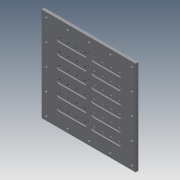
# Autodesk Inventor part: plate
Saved by Autodesk Inventor 2016 (Build 200138000, 138)
## iProperties
Created: 2013-02-21
Part Number: plate
Material: Generic
Document SubType Name: Modeling
Designer: Dave
Density: 1 g/cm^3
Appearance: Default
Author: Dave
Autodesk Inventor part; units mm, degrees
ref_plane "YZ Plane" through (0, 0, 0) normal (1, 0, 0) x (0, 1, 0)
ref_plane "XZ Plane" through (0, 0, 0) normal (0, 1, 0) x (-1, 0, 0)
ref_plane "XY Plane" through (0, 0, 0) normal (0, 0, 1) x (1, 0, 0)
sketch "Sketch1" plane through (0, 0, 0) normal (0, 0, 1) x (1, 0, 0)
  line L0 (0, 0) -> (219.964, 0)
  line L1 (219.964, 0) -> (219.964, 219.964)
  line L2 (219.964, 219.964) -> (0, 219.964)
  line L3 (0, 219.964) -> (0, 0)
  dimension "d0" = 219.964
  dimension "d1" = 219.964
  constraints: 8 end point, 2 parallel, 1 horizontal, 1 perpendicular
  measures "d0" distance of L0.start L0.end
  measures "d1" distance of L2.end L0.start
extrude "Plate" add sketch "Sketch1" along normal blind 6.5532
sketch "Sketch6" plane through (0, 0, 6.5532) normal (0, 0, 1) x (1, 0, 0)
  line L0 (0, 0) -> (0, 219.964) projected
  line L1 (219.964, 0) -> (0, 0) projected
  line L2 (219.964, 219.964) -> (219.964, 0) projected
  line L3 (0, 219.964) -> (219.964, 219.964) projected
  circle A0 centre (10.16, 209.804) radius 4.421
  circle A1 centre (60.071, 209.804) radius 4.421
  circle A2 centre (109.982, 209.804) radius 4.421
  circle A3 centre (159.893, 209.804) radius 4.421
  circle A4 centre (209.804, 209.804) radius 4.421
  circle A5 centre (10.16, 159.893) radius 4.421
  circle A6 centre (10.16, 109.982) radius 4.421
  circle A7 centre (10.16, 60.071) radius 4.421
  circle A8 centre (10.16, 10.16) radius 4.421
  circle A9 centre (60.071, 10.16) radius 4.421
  circle A10 centre (109.982, 10.16) radius 4.421
  circle A11 centre (159.893, 10.16) radius 4.421
  circle A12 centre (209.804, 10.16) radius 4.421
  circle A13 centre (209.804, 159.893) radius 4.421
  circle A14 centre (209.804, 109.982) radius 4.421
  circle A15 centre (209.804, 60.071) radius 4.421
  circle A16 centre (209.804, 10.16) radius 4.421
  dimension "d56" = 10.16
  dimension "d58" = 10.16
  dimension "d61" = 49.911
  dimension "d68" = 49.911
  dimension "d75" = 49.911
  dimension "d82" = 49.911
  constraints: 17 centre point, 2 horizontal, 2 vertical, 32 other
  measures "d56" distance from line of A0.centre L3
  measures "d58" distance from line of A0.centre L0
  measures "d61" distance of A0.centre A1.centre
  measures "d68" distance of A0.centre A5.centre
  measures "d75" distance of A8.centre A9.centre
  measures "d82" distance of A4.centre A13.centre
hole "Boundary" at (10.16, 209.804, 6.5532) at (60.071, 209.804, 6.5532) at (10.16, 159.893, 6.5532) at (109.982, 209.804, 6.5532) at (10.16, 109.982, 6.5532) at (159.893, 209.804, 6.5532) at (10.16, 60.071, 6.5532) at (209.804, 209.804, 6.5532) at (10.16, 10.16, 6.5532) at (209.804, 159.893, 6.5532) at (60.071, 10.16, 6.5532) at (209.804, 109.982, 6.5532) at (109.982, 10.16, 6.5532) at (209.804, 60.071, 6.5532) at (159.893, 10.16, 6.5532) at (209.804, 10.16, 6.5532) direction (0, 0, -1) diameter 6.35 end through all
sketch "Sketch10" plane through (0, 0, 6.5532) normal (0, 0, 1) x (1, 0, 0)
  circle A0 centre (10.16, 209.804) radius 3.175 projected
  line L0 (0, 0) -> (0, 219.964) projected
  line L1 (0, 219.964) -> (219.964, 219.964) projected
  circle A1 centre (40.4114, 179.5526) radius 3.175
  circle A2 centre (60.4012, 179.5526) radius 3.175
  circle A3 centre (80.391, 179.5526) radius 3.175
  circle A4 centre (100.3808, 179.5526) radius 3.175
  circle A5 centre (120.3706, 179.5526) radius 3.175
  circle A6 centre (140.3604, 179.5526) radius 3.175
  circle A7 centre (160.3502, 179.5526) radius 3.175
  circle A8 centre (180.34, 179.5526) radius 3.175
  circle A9 centre (40.4114, 151.5618) radius 3.175
  circle A10 centre (60.4012, 151.5618) radius 3.175
  circle A11 centre (80.391, 151.5618) radius 3.175
  circle A12 centre (100.3808, 151.5618) radius 3.175
  circle A13 centre (120.3706, 151.5618) radius 3.175
  circle A14 centre (140.3604, 151.5618) radius 3.175
  circle A15 centre (160.3502, 151.5618) radius 3.175
  circle A16 centre (180.34, 151.5618) radius 3.175
  circle A17 centre (40.4114, 123.571) radius 3.175
  circle A18 centre (60.4012, 123.571) radius 3.175
  circle A19 centre (80.391, 123.571) radius 3.175
  circle A20 centre (100.3808, 123.571) radius 3.175
  circle A21 centre (120.3706, 123.571) radius 3.175
  circle A22 centre (140.3604, 123.571) radius 3.175
  circle A23 centre (160.3502, 123.571) radius 3.175
  circle A24 centre (180.34, 123.571) radius 3.175
  circle A25 centre (40.4114, 95.5802) radius 3.175
  circle A26 centre (60.4012, 95.5802) radius 3.175
  circle A27 centre (80.391, 95.5802) radius 3.175
  circle A28 centre (100.3808, 95.5802) radius 3.175
  circle A29 centre (120.3706, 95.5802) radius 3.175
  circle A30 centre (140.3604, 95.5802) radius 3.175
  circle A31 centre (160.3502, 95.5802) radius 3.175
  circle A32 centre (180.34, 95.5802) radius 3.175
  circle A33 centre (40.4114, 67.5894) radius 3.175
  circle A34 centre (60.4012, 67.5894) radius 3.175
  circle A35 centre (80.391, 67.5894) radius 3.175
  circle A36 centre (100.3808, 67.5894) radius 3.175
  circle A37 centre (120.3706, 67.5894) radius 3.175
  circle A38 centre (140.3604, 67.5894) radius 3.175
  circle A39 centre (160.3502, 67.5894) radius 3.175
  circle A40 centre (180.34, 67.5894) radius 3.175
  circle A41 centre (40.4114, 39.5986) radius 3.175
  circle A42 centre (60.4012, 39.5986) radius 3.175
  circle A43 centre (80.391, 39.5986) radius 3.175
  circle A44 centre (100.3808, 39.5986) radius 3.175
  circle A45 centre (120.3706, 39.5986) radius 3.175
  circle A46 centre (140.3604, 39.5986) radius 3.175
  circle A47 centre (160.3502, 39.5986) radius 3.175
  circle A48 centre (180.34, 39.5986) radius 3.175
  dimension "d175" = 6.35
  dimension "d177" = 30.2514
  dimension "d178" = 30.2514
  dimension "d181" = 19.9898
  dimension "d184" = 27.9908
  constraints: 48 centre point, 1 horizontal, 1 vertical, 94 other
  measures "d175" diameter of A1
  measures "d177" horizontal distance of A0.centre A1.centre
  measures "d178" horizontal distance of A1.centre A0.centre
  measures "d181" distance of A1.centre A2.centre
  measures "d184" distance of A1.centre A9.centre
hole "SMA" at (80.391, 123.571, 6.5532) at (100.3808, 123.571, 6.5532) at (80.391, 151.5618, 6.5532) at (100.3808, 151.5618, 6.5532) at (80.391, 179.5526, 6.5532) at (100.3808, 179.5526, 6.5532) at (60.4012, 151.5618, 6.5532) at (40.4114, 151.5618, 6.5532) at (40.4114, 179.5526, 6.5532) at (60.4012, 179.5526, 6.5532) at (40.4114, 123.571, 6.5532) at (60.4012, 123.571, 6.5532) at (40.4114, 95.5802, 6.5532) at (60.4012, 95.5802, 6.5532) at (80.391, 95.5802, 6.5532) at (100.3808, 67.5894, 6.5532) at (80.391, 67.5894, 6.5532) at (80.391, 39.5986, 6.5532) at (60.4012, 67.5894, 6.5532) at (60.4012, 39.5986, 6.5532) at (40.4114, 39.5986, 6.5532) at (40.4114, 67.5894, 6.5532) at (100.3808, 95.5802, 6.5532) at (120.3706, 179.5526, 6.5532) at (140.3604, 179.5526, 6.5532) at (160.3502, 179.5526, 6.5532) at (180.34, 179.5526, 6.5532) at (120.3706, 151.5618, 6.5532) at (140.3604, 151.5618, 6.5532) at (120.3706, 95.5802, 6.5532) at (140.3604, 123.571, 6.5532) at (140.3604, 95.5802, 6.5532) at (160.3502, 151.5618, 6.5532) at (160.3502, 123.571, 6.5532) at (180.34, 151.5618, 6.5532) at (160.3502, 95.5802, 6.5532) at (180.34, 123.571, 6.5532) at (180.34, 95.5802, 6.5532) at (120.3706, 123.571, 6.5532) at (100.3808, 39.5986, 6.5532) at (120.3706, 67.5894, 6.5532) at (120.3706, 39.5986, 6.5532) at (140.3604, 67.5894, 6.5532) at (140.3604, 39.5986, 6.5532) at (160.3502, 67.5894, 6.5532) at (160.3502, 39.5986, 6.5532) at (180.34, 67.5894, 6.5532) at (180.34, 39.5986, 6.5532) direction (0, 0, -1) diameter 5.588 end through all thread size "1/4-36 UNS" class "2B" standard "ANSI Unified Screw Threads"
sketch "Sketch12" plane through (0, 0, 6.5532) normal (0, 0, 1) x (1, 0, 0)
  circle A0 centre (40.4114, 179.5526) radius 2.794 projected
  circle A1 centre (80.391, 179.5526) radius 2.794 projected
  circle A2 centre (100.3808, 179.5526) radius 2.794 projected
  circle A3 centre (60.4012, 179.5526) radius 2.794 projected
  arc A4 (40.4114, 185.9026) -> (40.4114, 173.2026) centre (40.4114, 179.5526) ccw
  arc A5 (100.3808, 173.2026) -> (100.3808, 185.9026) centre (100.3808, 179.5526) ccw
  line L0 (40.4114, 185.9026) -> (100.3808, 185.9026)
  line L1 (40.4114, 173.2026) -> (100.3808, 173.2026)
  dimension "d211" = 12.7
  dimension "d213" = 12.7
  constraints: 4 end point, 4 point on circle, 2 centre point, 2 coincident, 2 tangent, 1 parallel
  measures "d211" diameter of A4
  measures "d213" diameter of A5
extrude "Extrusion3" cut sketch "Sketch12" against normal blind 2.667
pattern_linear "Rectangular Pattern1" count 2 spacing 80.01 along (1, 0, 0) count 6 spacing 27.9908 along (0, -1, 0) of "Extrusion3"
sketch "Sketch11" plane through (0, 0, 6.5532) normal (0, 0, 1) x (1, 0, 0)
  circle A0 centre (40.4114, 179.5526) radius 2.794 projected
  line L0 (0, 0) -> (0, 219.964) projected
  line L1 (0, 219.964) -> (219.964, 219.964) projected
  circle A1 centre (31.5214, 188.4426) radius 2.4311
  circle A2 centre (110.2614, 188.4426) radius 2.4311
  circle A3 centre (189.0014, 188.4426) radius 2.4311
  circle A4 centre (31.5214, 160.4518) radius 2.4311
  circle A5 centre (110.2614, 160.4518) radius 2.4311
  circle A6 centre (189.0014, 160.4518) radius 2.4311
  circle A7 centre (31.5214, 132.461) radius 2.4311
  circle A8 centre (110.2614, 132.461) radius 2.4311
  circle A9 centre (189.0014, 132.461) radius 2.4311
  circle A10 centre (31.5214, 104.4702) radius 2.4311
  circle A11 centre (110.2614, 104.4702) radius 2.4311
  circle A12 centre (189.0014, 104.4702) radius 2.4311
  circle A13 centre (31.5214, 76.4794) radius 2.4311
  circle A14 centre (110.2614, 76.4794) radius 2.4311
  circle A15 centre (189.0014, 76.4794) radius 2.4311
  circle A16 centre (31.5214, 48.4886) radius 2.4311
  circle A17 centre (110.2614, 48.4886) radius 2.4311
  circle A18 centre (189.0014, 48.4886) radius 2.4311
  dimension "d194" = 8.89
  dimension "d195" = 8.89
  dimension "d198" = 78.74
  dimension "d201" = 27.9908
  constraints: 18 centre point, 1 horizontal, 1 vertical, 34 other
  measures "d194" horizontal distance of A0.centre A1.centre
  measures "d195" horizontal distance of A1.centre A0.centre
  measures "d198" distance of A1.centre A2.centre
  measures "d201" distance of A1.centre A4.centre
hole "Hole12" at (31.5214, 188.4426, 6.5532) at (31.5214, 160.4518, 6.5532) at (31.5214, 132.461, 6.5532) at (31.5214, 104.4702, 6.5532) at (31.5214, 76.4794, 6.5532) at (31.5214, 48.4886, 6.5532) at (110.2614, 188.4426, 6.5532) at (110.2614, 104.4702, 6.5532) at (110.2614, 160.4518, 6.5532) at (110.2614, 132.461, 6.5532) at (110.2614, 76.4794, 6.5532) at (110.2614, 48.4886, 6.5532) at (189.0014, 132.461, 6.5532) at (189.0014, 160.4518, 6.5532) at (189.0014, 188.4426, 6.5532) at (189.0014, 104.4702, 6.5532) at (189.0014, 76.4794, 6.5532) at (189.0014, 48.4886, 6.5532) direction (0, 0, -1) diameter 3.2512 end through all
body "Solid1"
